Autodesk Fusion 360 part; units mm, degrees
(part 3 of 5)
  line L278 (101.5867, -7.7448) -> (99.4171, -13.4118)
  line L279 (99.4171, -13.4118) -> (84.4237, -13.4118)
  line L280 (84.4237, -13.4118) -> (91.9366, 2.5207)
  line L281 (97.7331, -10.8212) -> (98.057, -10.044)
  line L282 (98.057, -10.044) -> (90.1879, -10.044)
  line L283 (90.1879, -10.044) -> (97.5712, 5.5971)
  line L284 (97.5712, 5.5971) -> (89.864, 5.5971)
  line L285 (89.864, 5.5971) -> (89.5726, 4.8199)
  line L286 (89.5726, 4.8199) -> (96.2435, 4.8199)
  line L287 (96.2435, 4.8199) -> (88.8602, -10.8212)
  line L288 (88.8602, -10.8212) -> (97.7331, -10.8212)
extrude "Extrude1" add sketch "Sketch1" along normal blind 2 contours S0 S1 S2 L0 S3 S5 S6 L2 S7 S8 S9 S10 S11 L3 S12 S13 S14 S15 S16 S17 S18 S19 S20 S21 S22 S46 | S3 L1 S4 S5 S34 S35 S36 S37 S40 S41 S42 S43 S44 S45 S46 S47 S48 S49 S50 L5 S51 S52 S53 S54 L6 S55 S56 S57 S64 | S3 L1 S4 S5 S46 | S37 S38 S39 S40 S64 | S37 S38 S39 S40 L7 S58 S59 S60 S61 S62 S63 L8 S64 S65 S66 L9 S67 S68 S69 S70 S71 S72 S73 S74 S75 S77 S78 S79 S83 | S75 S76 S77 S83 | S75 S76 S77 S80 S81 S82 S83 S84 S85 S86 S87 S88 S89 S90 S91 S92 S93 S98 S134 S135 | S93 S94 S95 S96 S97 S98 S134 S135 | S93 S94 S95 S96 S97 S98 S106 S107 S108 S109 S110 S111 S112 S113 S114 S115 S116 S117 S118 S119 S120 S121 S122 S123 S124 S125 S126 S127 S128 S129 S130 S131 S132 S133 S134 S135 S136 S137 S138 S139 S140 S141 S142 S143 | L11 S148 S149 S150 S151 S152 L12 S153 S154 S155 S156 S157 S158 L13 S159 S160 S161 S162 S163 S164 L14 S165 S166 S167 S168 S169 S170 | S400 S401 S402 S403 S404 S405 S406 S407 S408 S409 S410 S411 S412 L177 S413 S414 S415 S416 L178 | S417 S418 L179 S419 S420 S421 L180 S422 S423 L181 S424 S425 S426 S427 S428 S429 S430 S431 S432 S433 S434 L182 S435 S436 S437 L183 S438 S439 L184 S440 | S441 S442 S443 L185 S444 S445 S446 S447 S448 S449 S450 S451 S452 S453 S454 L186 S455 S456 S457 S458 S459 L187 S460 S461 S462 S463 L188 S464 S465 S466 S467 S468 S469 S470 S471 S472 L189 | S473 S474 S475 L190 S476 S477 S478 S479 S480 S481 S482 S483 S484 S485 S486 S487 S488 S489 S490 S491 S492 S493 S494 S495 S496 S497 S498 L191 | S504 L192 S505 S506 L193 S507 S508 S509 S510 S511 S512 S513 S514 S515 S516 S517 S518 S519 S520 L194 S521 S522 S523 S524 S525 S526 S527 S528 S529 S530 S531 | S532 S533 S534 S535 S536 S537 S538 S539 L195 S540 S541 S542 S543 L196 S544 S545 S546 S547 S548 S549 S550 L197 S551 S552 S553 L198 S554 | L199 S555 S556 L200 L201 L202 S557 S558 L203 L204 | S563 S564 S565 S566 L211 L212 L213 S567 S568 S569 S570 L214 L215 L216 S571 S572 S573 S574 | L223 L224 L225 L226 L227 L228 L229 L230 L231 L232 L233 L234 | L247 L248 L249 L250 L251 L252 L253 L254 S650 L272 | L248 S614 S615 S616 S617 S618 S619 S620 S621 S622 S623 S624 S625 S626 S627 S628 S629 S630 L271 S631 S632 S633 S634 S635 S636 S637 S638 S639 S640 S641 S642 S643 S644 S645 S646 S647 S648 S649 S650 L272 | L248 S650 L272 | L266 L267 L268 | L273 L274 L275 L276 L277 L278 L279 L280 makes body 1 at (67.0712, -5.2622, 0) makes body 2 at (83.8602, -73.7685, 0) makes body 3 at (35.5259, -74.9694, 0) makes body 4 at (11.5017, -77.2089, 0) makes body 5 at (12.3957, 2.7474, 0) makes body 6 at (94.6365, -86.6871, 0) makes body 7 at (28.3473, -77.0944, 0) makes body 8 at (63.6816, -78.7236, 0) makes body 9 at (34.5713, 94.918, 0) makes body 10 at (90.4627, 77.2296, 0) makes body 11 at (98.0246, 2.0134, 0) makes body 12 at (8.1997, 1.9486, 0) makes body 13 at (62.0414, -2.1749, 0) makes body 14 at (32.4794, 0.1243, 0)
sketch "Sketch2" plane through (0, 0, 0) normal (0, 0, 1) x (1, 0, 0)
  spline S0 degree 3 poles (-205.111, 36.7973) (-205.4906, 36.9633) (-205.8582, 37.0464) (-206.214, 37.0464) knots 0 0 0 0 1 1 1 1
  spline S1 degree 3 poles (-206.214, 37.0464) (-206.5698, 37.0464) (-206.9256, 36.821) (-207.2814, 36.3703) knots 0 0 0 0 1 1 1 1
  spline S2 degree 3 poles (-207.2814, 36.3703) (-207.6372, 35.9197) (-207.8744, 35.2674) (-207.993, 34.4135) knots 0 0 0 0 1 1 1 1
  line L0 (-207.993, 34.4135) -> (-209.7719, 21.9608)
  spline S3 degree 3 poles (-209.7719, 21.9608) (-206.7833, 23.2653) (-204.8738, 24.2378) (-204.0437, 24.8783) knots 0 0 0 0 1 1 1 1
  line L1 (-204.0437, 24.8783) -> (-202.6916, 22.53)
  spline S4 degree 3 poles (-202.6916, 22.53) (-203.4032, 21.9845) (-204.2571, 21.4982) (-205.2534, 21.0713) knots 0 0 0 0 1 1 1 1
  spline S5 degree 3 poles (-205.2534, 21.0713) (-206.2496, 20.6443) (-207.2102, 20.2411) (-208.1353, 19.8616) knots 0 0 0 0 1 1 1 1
  spline S6 degree 3 poles (-208.1353, 19.8616) (-209.0603, 19.5058) (-209.7482, 19.233) (-210.1989, 19.0433) knots 0 0 0 0 1 1 1 1
  line L2 (-210.1989, 19.0433) -> (-211.373, 10.7177)
  spline S7 degree 3 poles (-211.373, 10.7177) (-211.6813, 8.4407) (-212.4997, 6.7684) (-213.8279, 5.7011) knots 0 0 0 0 1 1 1 1
  spline S8 degree 3 poles (-213.8279, 5.7011) (-215.1325, 4.6099) (-216.5794, 4.0644) (-218.1686, 4.0644) knots 0 0 0 0 1 1 1 1
  spline S9 degree 3 poles (-218.1686, 4.0644) (-219.7341, 4.0644) (-220.9794, 4.6455) (-221.9044, 5.8078) knots 0 0 0 0 1 1 1 1
  spline S10 degree 3 poles (-221.9044, 5.8078) (-222.8295, 6.9463) (-223.292, 8.2272) (-223.292, 9.6504) knots 0 0 0 0 1 1 1 1
  spline S11 degree 3 poles (-223.292, 9.6504) (-223.292, 13.3743) (-220.5643, 16.6832) (-215.1088, 19.5769) knots 0 0 0 0 1 1 1 1
  line L3 (-215.1088, 19.5769) -> (-214.753, 22.4589)
  spline S12 degree 3 poles (-214.753, 22.4589) (-214.3023, 26.5386) (-213.8398, 30.0847) (-213.3654, 33.097) knots 0 0 0 0 1 1 1 1
  spline S13 degree 3 poles (-213.3654, 33.097) (-214.7174, 32.5515) (-216.1406, 32.2787) (-217.6349, 32.2787) knots 0 0 0 0 1 1 1 1
  spline S14 degree 3 poles (-217.6349, 32.2787) (-219.1055, 32.2787) (-220.3034, 32.682) (-221.2284, 33.4884) knots 0 0 0 0 1 1 1 1
  spline S15 degree 3 poles (-221.2284, 33.4884) (-222.1298, 34.2949) (-222.5804, 35.3504) (-222.5804, 36.655) knots 0 0 0 0 1 1 1 1
  spline S16 degree 3 poles (-222.5804, 36.655) (-222.5804, 37.9596) (-222.1179, 38.9795) (-221.1928, 39.7148) knots 0 0 0 0 1 1 1 1
  spline S17 degree 3 poles (-221.1928, 39.7148) (-220.2441, 40.4738) (-219.0581, 40.8533) (-217.6349, 40.8533) knots 0 0 0 0 1 1 1 1
  spline S18 degree 3 poles (-217.6349, 40.8533) (-216.7573, 40.8533) (-215.5002, 40.5806) (-213.8635, 40.035) knots 0 0 0 0 1 1 1 1
  spline S19 degree 3 poles (-213.8635, 40.035) (-212.2031, 39.4895) (-210.9223, 39.2167) (-210.021, 39.2167) knots 0 0 0 0 1 1 1 1
  spline S20 degree 3 poles (-210.021, 39.2167) (-208.4081, 39.2167) (-207.056, 39.6318) (-205.9649, 40.462) knots 0 0 0 0 1 1 1 1
  spline S21 degree 3 poles (-205.9649, 40.462) (-205.3719, 39.6318) (-205.0755, 38.6474) (-205.0755, 37.5089) knots 0 0 0 0 1 1 1 1
  spline S22 degree 3 poles (-205.0755, 37.5089) (-205.0755, 37.2717) (-205.0873, 37.0345) (-205.111, 36.7973) knots 0 0 0 0 1 1 1 1
  spline S23 degree 3 poles (-219.0581, 35.6943) (-219.0581, 35.3385) (-218.8683, 35.0302) (-218.4888, 34.7693) knots 0 0 0 0 1 1 1 1
  spline S24 degree 3 poles (-218.4888, 34.7693) (-218.0856, 34.5084) (-217.4926, 34.3779) (-216.7099, 34.3779) knots 0 0 0 0 1 1 1 1
  spline S25 degree 3 poles (-216.7099, 34.3779) (-215.9034, 34.3779) (-214.8597, 34.7337) (-213.5789, 35.4453) knots 0 0 0 0 1 1 1 1
  spline S26 degree 3 poles (-213.5789, 35.4453) (-214.5039, 35.6588) (-215.4527, 35.896) (-216.4252, 36.1569) knots 0 0 0 0 1 1 1 1
  spline S27 degree 3 poles (-216.4252, 36.1569) (-217.3977, 36.4415) (-217.9789, 36.5838) (-218.1686, 36.5838) knots 0 0 0 0 1 1 1 1
  spline S28 degree 3 poles (-218.1686, 36.5838) (-218.7616, 36.5838) (-219.0581, 36.2873) (-219.0581, 35.6943) knots 0 0 0 0 1 1 1 1
  spline S29 degree 3 poles (-215.5002, 16.4816) (-218.892, 14.4417) (-220.588, 12.2832) (-220.588, 10.0061) knots 0 0 0 0 1 1 1 1
  spline S30 degree 3 poles (-220.588, 10.0061) (-220.588, 9.3657) (-220.422, 8.8202) (-220.0899, 8.3695) knots 0 0 0 0 1 1 1 1
  spline S31 degree 3 poles (-220.0899, 8.3695) (-219.7104, 7.8477) (-219.236, 7.5868) (-218.6667, 7.5868) knots 0 0 0 0 1 1 1 1
  spline S32 degree 3 poles (-218.6667, 7.5868) (-218.0737, 7.5868) (-217.5638, 7.7647) (-217.1368, 8.1204) knots 0 0 0 0 1 1 1 1
  spline S33 degree 3 poles (-217.1368, 8.1204) (-216.7099, 8.4762) (-216.449, 9.0455) (-216.3541, 9.8282) knots 0 0 0 0 1 1 1 1
  line L4 (-216.3541, 9.8282) -> (-215.5002, 16.4816)
  spline S34 degree 3 poles (-191.4142, 30.5709) (-192.3866, 22.8858) (-192.8729, 18.7942) (-192.8729, 18.2961) knots 0 0 0 0 1 1 1 1
  spline S35 degree 3 poles (-192.8729, 18.2961) (-192.8729, 17.3474) (-192.529, 16.8729) (-191.8411, 16.8729) knots 0 0 0 0 1 1 1 1
  spline S36 degree 3 poles (-191.8411, 16.8729) (-191.2244, 16.8729) (-190.5603, 17.288) (-189.8487, 18.1182) knots 0 0 0 0 1 1 1 1
  spline S37 degree 3 poles (-189.8487, 18.1182) (-189.1134, 18.9721) (-188.5322, 20.2411) (-188.1053, 21.9252) knots 0 0 0 0 1 1 1 1
  spline S38 degree 3 poles (-188.1053, 21.9252) (-187.3225, 21.0713) (-186.8481, 20.4071) (-186.6821, 19.9327) knots 0 0 0 0 1 1 1 1
  spline S39 degree 3 poles (-186.6821, 19.9327) (-187.2277, 17.6319) (-188.0934, 16.0072) (-189.2794, 15.0584) knots 0 0 0 0 1 1 1 1
  spline S40 degree 3 poles (-189.2794, 15.0584) (-190.4654, 14.1096) (-191.6869, 13.6352) (-192.9441, 13.6352) knots 0 0 0 0 1 1 1 1
  spline S41 degree 3 poles (-192.9441, 13.6352) (-195.0077, 13.6352) (-196.3952, 14.4298) (-197.1068, 16.019) knots 0 0 0 0 1 1 1 1
  spline S42 degree 3 poles (-197.1068, 16.019) (-198.3402, 14.4298) (-199.9887, 13.6352) (-202.0523, 13.6352) knots 0 0 0 0 1 1 1 1
  spline S43 degree 3 poles (-202.0523, 13.6352) (-203.7601, 13.6352) (-205.0766, 14.0622) (-206.0016, 14.9161) knots 0 0 0 0 1 1 1 1
  spline S44 degree 3 poles (-206.0016, 14.9161) (-206.9267, 15.77) (-207.3892, 16.8848) (-207.3892, 18.2605) knots 0 0 0 0 1 1 1 1
  spline S45 degree 3 poles (-207.3892, 18.2605) (-207.3892, 18.5926) (-207.3299, 19.1737) (-207.2113, 20.0039) knots 0 0 0 0 1 1 1 1
  spline S46 degree 3 poles (-207.2113, 20.0039) (-206.6657, 24.4157) (-206.2507, 27.9262) (-205.9661, 30.5353) knots 0 0 0 0 1 1 1 1
  spline S47 degree 3 poles (-205.9661, 30.5353) (-205.2307, 30.7963) (-204.5547, 30.9267) (-203.938, 30.9267) knots 0 0 0 0 1 1 1 1
  spline S48 degree 3 poles (-203.938, 30.9267) (-203.3213, 30.9267) (-202.8588, 30.903) (-202.5504, 30.8556) knots 0 0 0 0 1 1 1 1
  spline S49 degree 3 poles (-202.5504, 30.8556) (-202.2421, 30.8081) (-201.9456, 30.6302) (-201.661, 30.3219) knots 0 0 0 0 1 1 1 1
  spline S50 degree 3 poles (-201.661, 30.3219) (-201.3763, 30.0136) (-201.234, 29.5747) (-201.234, 29.0054) knots 0 0 0 0 1 1 1 1
  line L5 (-201.234, 29.0054) -> (-202.4081, 19.9327)
  spline S51 degree 3 poles (-202.4081, 19.9327) (-202.4556, 19.6481) (-202.4793, 19.3872) (-202.4793, 19.15) knots 0 0 0 0 1 1 1 1
  spline S52 degree 3 poles (-202.4793, 19.15) (-202.4793, 17.7506) (-201.8389, 17.0508) (-200.558, 17.0508) knots 0 0 0 0 1 1 1 1
  spline S53 degree 3 poles (-200.558, 17.0508) (-199.372, 17.0508) (-198.3877, 17.632) (-197.6049, 18.7942) knots 0 0 0 0 1 1 1 1
  spline S54 degree 3 poles (-197.6049, 18.7942) (-197.6049, 19.0552) (-197.5812, 19.4702) (-197.5338, 20.0395) knots 0 0 0 0 1 1 1 1
  line L6 (-197.5338, 20.0395) -> (-196.3597, 29.5035)
  spline S55 degree 3 poles (-196.3597, 29.5035) (-196.1936, 29.9068) (-195.8378, 30.2389) (-195.2923, 30.4998) knots 0 0 0 0 1 1 1 1
  spline S56 degree 3 poles (-195.2923, 30.4998) (-194.7467, 30.7844) (-194.0707, 30.9267) (-193.2643, 30.9267) knots 0 0 0 0 1 1 1 1
  spline S57 degree 3 poles (-193.2643, 30.9267) (-192.4341, 30.9267) (-191.8174, 30.8081) (-191.4142, 30.5709) knots 0 0 0 0 1 1 1 1
  line L7 (-179.5365, 17.8691) -> (-178.6826, 25.7322)
  spline S58 degree 3 poles (-178.6826, 25.7322) (-178.6826, 26.3726) (-178.8487, 26.9063) (-179.1808, 27.3332) knots 0 0 0 0 1 1 1 1
  spline S59 degree 3 poles (-179.1808, 27.3332) (-179.5128, 27.7602) (-180.0465, 27.9736) (-180.7818, 27.9736) knots 0 0 0 0 1 1 1 1
  spline S60 degree 3 poles (-180.7818, 27.9736) (-181.5171, 27.9736) (-182.1457, 27.6772) (-182.6675, 27.0842) knots 0 0 0 0 1 1 1 1
  spline S61 degree 3 poles (-182.6675, 27.0842) (-183.1656, 26.5149) (-183.5333, 25.7559) (-183.7705, 24.8071) knots 0 0 0 0 1 1 1 1
  spline S62 degree 3 poles (-183.7705, 24.8071) (-183.9365, 23.4551) (-184.1855, 21.4745) (-184.5176, 18.8654) knots 0 0 0 0 1 1 1 1
  spline S63 degree 3 poles (-184.5176, 18.8654) (-184.8497, 16.28) (-185.0632, 14.5959) (-185.1581, 13.8131) knots 0 0 0 0 1 1 1 1
  line L8 (-185.1581, 13.8131) -> (-189.8901, 13.8131)
  spline S64 degree 3 poles (-189.8901, 13.8131) (-188.1823, 28.3532) (-187.1505, 37.2835) (-186.7947, 40.6043) knots 0 0 0 0 1 1 1 1
  spline S65 degree 3 poles (-186.7947, 40.6043) (-186.2966, 40.794) (-185.6206, 40.8889) (-184.7667, 40.8889) knots 0 0 0 0 1 1 1 1
  spline S66 degree 3 poles (-184.7667, 40.8889) (-182.9166, 40.8889) (-181.9915, 40.3434) (-181.9915, 39.2523) knots 0 0 0 0 1 1 1 1
  line L9 (-181.9915, 39.2523) -> (-181.9915, 39.0388)
  spline S67 degree 3 poles (-181.9915, 39.0388) (-182.3947, 35.3149) (-182.8217, 32.0416) (-183.2724, 29.2189) knots 0 0 0 0 1 1 1 1
  spline S68 degree 3 poles (-183.2724, 29.2189) (-182.0152, 30.3574) (-180.592, 30.9267) (-179.0029, 30.9267) knots 0 0 0 0 1 1 1 1
  spline S69 degree 3 poles (-179.0029, 30.9267) (-177.4136, 30.9267) (-176.1565, 30.5235) (-175.2315, 29.717) knots 0 0 0 0 1 1 1 1
  spline S70 degree 3 poles (-175.2315, 29.717) (-174.3064, 28.9106) (-173.8439, 27.8906) (-173.8439, 26.6572) knots 0 0 0 0 1 1 1 1
  spline S71 degree 3 poles (-173.8439, 26.6572) (-173.8439, 26.3252) (-173.915, 25.7085) (-174.0573, 24.8071) knots 0 0 0 0 1 1 1 1
  spline S72 degree 3 poles (-174.0573, 24.8071) (-174.6029, 21.2492) (-174.8757, 19.1619) (-174.8757, 18.5452) knots 0 0 0 0 1 1 1 1
  spline S73 degree 3 poles (-174.8757, 18.5452) (-174.8757, 17.4304) (-174.508, 16.8729) (-173.7727, 16.8729) knots 0 0 0 0 1 1 1 1
  spline S74 degree 3 poles (-173.7727, 16.8729) (-173.156, 16.8729) (-172.5037, 17.2762) (-171.816, 18.0826) knots 0 0 0 0 1 1 1 1
  spline S75 degree 3 poles (-171.816, 18.0826) (-171.1044, 18.9128) (-170.5352, 20.1818) (-170.1082, 21.8896) knots 0 0 0 0 1 1 1 1
  spline S76 degree 3 poles (-170.1082, 21.8896) (-169.3016, 21.0357) (-168.8152, 20.3597) (-168.6495, 19.8616) knots 0 0 0 0 1 1 1 1
  spline S77 degree 3 poles (-168.6495, 19.8616) (-169.8825, 15.7344) (-172.0651, 13.6708) (-175.1959, 13.6708) knots 0 0 0 0 1 1 1 1
  spline S78 degree 3 poles (-175.1959, 13.6708) (-176.6665, 13.6708) (-177.7576, 14.1215) (-178.4692, 15.0228) knots 0 0 0 0 1 1 1 1
  spline S79 degree 3 poles (-178.4692, 15.0228) (-179.1808, 15.9241) (-179.5365, 16.8729) (-179.5365, 17.8691) knots 0 0 0 0 1 1 1 1
  spline S80 degree 3 poles (-155.7317, 13.6352) (-157.9137, 13.6352) (-159.3607, 14.3942) (-160.0723, 15.9123) knots 0 0 0 0 1 1 1 1
  spline S81 degree 3 poles (-160.0723, 15.9123) (-161.3054, 14.3705) (-162.8948, 13.5996) (-164.8399, 13.5996) knots 0 0 0 0 1 1 1 1
  spline S82 degree 3 poles (-164.8399, 13.5996) (-166.7612, 13.5996) (-168.3857, 14.2519) (-169.7143, 15.5565) knots 0 0 0 0 1 1 1 1
  spline S83 degree 3 poles (-169.7143, 15.5565) (-171.0185, 16.8611) (-171.6712, 18.5807) (-171.6712, 20.7155) knots 0 0 0 0 1 1 1 1
  spline S84 degree 3 poles (-171.6712, 20.7155) (-171.6712, 23.8228) (-170.7578, 26.3014) (-168.9316, 28.1515) knots 0 0 0 0 1 1 1 1
  spline S85 degree 3 poles (-168.9316, 28.1515) (-167.1048, 30.0017) (-164.7922, 30.9267) (-161.9936, 30.9267) knots 0 0 0 0 1 1 1 1
  spline S86 degree 3 poles (-161.9936, 30.9267) (-161.9225, 30.9267) (-161.8513, 30.9267) (-161.7801, 30.9267) knots 0 0 0 0 1 1 1 1
  spline S87 degree 3 poles (-161.7801, 30.9267) (-160.5938, 30.9267) (-159.5031, 30.7251) (-158.5068, 30.3219) knots 0 0 0 0 1 1 1 1
  spline S88 degree 3 poles (-158.5068, 30.3219) (-157.8664, 30.7251) (-157.0954, 30.9267) (-156.1942, 30.9267) knots 0 0 0 0 1 1 1 1
  spline S89 degree 3 poles (-156.1942, 30.9267) (-155.2691, 30.9267) (-154.6048, 30.8081) (-154.2018, 30.5709) knots 0 0 0 0 1 1 1 1
  spline S90 degree 3 poles (-154.2018, 30.5709) (-154.4152, 28.8157) (-154.6404, 27.0842) (-154.8778, 25.3764) knots 0 0 0 0 1 1 1 1
  spline S91 degree 3 poles (-154.8778, 25.3764) (-155.1146, 23.6923) (-155.2808, 22.4944) (-155.3759, 21.7829) knots 0 0 0 0 1 1 1 1
  spline S92 degree 3 poles (-155.3759, 21.7829) (-155.5894, 20.17) (-155.6961, 19.0077) (-155.6961, 18.2961) knots 0 0 0 0 1 1 1 1
  spline S93 degree 3 poles (-155.6961, 18.2961) (-155.6961, 17.3474) (-155.3164, 16.8729) (-154.5576, 16.8729) knots 0 0 0 0 1 1 1 1
  spline S94 degree 3 poles (-154.5576, 16.8729) (-153.9644, 16.8729) (-153.3357, 17.2643) (-152.6719, 18.047) knots 0 0 0 0 1 1 1 1
  spline S95 degree 3 poles (-152.6719, 18.047) (-152.0075, 18.8535) (-151.4266, 20.1106) (-150.9285, 21.8184) knots 0 0 0 0 1 1 1 1
  spline S96 degree 3 poles (-150.9285, 21.8184) (-150.2403, 21.2018) (-149.7661, 20.5139) (-149.5053, 19.7548) knots 0 0 0 0 1 1 1 1
  spline S97 degree 3 poles (-149.5053, 19.7548) (-150.193, 17.5015) (-151.1181, 15.9123) (-152.2805, 14.9872) knots 0 0 0 0 1 1 1 1
  spline S98 degree 3 poles (-152.2805, 14.9872) (-153.4424, 14.0859) (-154.5931, 13.6352) (-155.7317, 13.6352) knots 0 0 0 0 1 1 1 1
  spline S99 degree 3 poles (-161.4599, 28.1515) (-162.9776, 28.1515) (-164.1873, 27.5704) (-165.089, 26.4082) knots 0 0 0 0 1 1 1 1
  spline S100 degree 3 poles (-165.089, 26.4082) (-165.9663, 25.2696) (-166.4883, 23.5618) (-166.6545, 21.2848) knots 0 0 0 0 1 1 1 1
  spline S101 degree 3 poles (-166.6545, 21.2848) (-166.6779, 21.0713) (-166.6901, 20.8697) (-166.6901, 20.6799) knots 0 0 0 0 1 1 1 1
  spline S102 degree 3 poles (-166.6901, 20.6799) (-166.6901, 19.5177) (-166.4171, 18.5926) (-165.8717, 17.9047) knots 0 0 0 0 1 1 1 1
  spline S103 degree 3 poles (-165.8717, 17.9047) (-165.3025, 17.2169) (-164.5787, 16.8729) (-163.7014, 16.8729) knots 0 0 0 0 1 1 1 1
  spline S104 degree 3 poles (-163.7014, 16.8729) (-162.2071, 16.8729) (-161.0802, 17.9285) (-160.3214, 20.0395) knots 0 0 0 0 1 1 1 1
  line L10 (-160.3214, 20.0395) -> (-159.4675, 27.7246)
  spline S105 degree 3 poles (-159.4675, 27.7246) (-160.1552, 28.0092) (-160.8195, 28.1515) (-161.4599, 28.1515) knots 0 0 0 0 1 1 1 1
  spline S106 degree 3 poles (-137.2, 24.7004) (-135.326, 23.3247) (-134.3892, 21.6999) (-134.3892, 19.826) knots 0 0 0 0 1 1 1 1
  spline S107 degree 3 poles (-134.3892, 19.826) (-134.3892, 17.9521) (-135.1247, 16.446) (-136.5951, 15.3074) knots 0 0 0 0 1 1 1 1
  spline S108 degree 3 poles (-136.5951, 15.3074) (-138.0656, 14.1689) (-139.9157, 13.5996) (-142.1455, 13.5996) knots 0 0 0 0 1 1 1 1
  spline S109 degree 3 poles (-142.1455, 13.5996) (-143.5926, 13.5996) (-144.8022, 13.9554) (-145.7746, 14.667) knots 0 0 0 0 1 1 1 1
  spline S110 degree 3 poles (-145.7746, 14.667) (-146.7235, 15.4023) (-147.1977, 16.3037) (-147.1977, 17.371) knots 0 0 0 0 1 1 1 1
  spline S111 degree 3 poles (-147.1977, 17.371) (-147.1977, 18.4384) (-146.8419, 19.2805) (-146.1304, 19.8972) knots 0 0 0 0 1 1 1 1
  spline S112 degree 3 poles (-146.1304, 19.8972) (-145.4188, 20.5376) (-144.5293, 20.929) (-143.4619, 21.0713) knots 0 0 0 0 1 1 1 1
  spline S113 degree 3 poles (-143.4619, 21.0713) (-143.96, 20.3597) (-144.2091, 19.6718) (-144.2091, 19.0077) knots 0 0 0 0 1 1 1 1
  spline S114 degree 3 poles (-144.2091, 19.0077) (-144.2091, 18.3673) (-143.9839, 17.8455) (-143.5331, 17.4422) knots 0 0 0 0 1 1 1 1
  spline S115 degree 3 poles (-143.5331, 17.4422) (-143.0822, 17.039) (-142.513, 16.8374) (-141.8253, 16.8374) knots 0 0 0 0 1 1 1 1
  spline S116 degree 3 poles (-141.8253, 16.8374) (-141.1376, 16.8374) (-140.5683, 17.0864) (-140.1175, 17.5845) knots 0 0 0 0 1 1 1 1
  spline S117 degree 3 poles (-140.1175, 17.5845) (-139.6666, 18.1064) (-139.4415, 18.6994) (-139.4415, 19.3635) knots 0 0 0 0 1 1 1 1
  spline S118 degree 3 poles (-139.4415, 19.3635) (-139.4415, 20.4546) (-139.9513, 21.4271) (-140.9714, 22.281) knots 0 0 0 0 1 1 1 1
  spline S119 degree 3 poles (-140.9714, 22.281) (-141.5879, 22.7791) (-142.2522, 23.2416) (-142.9638, 23.6686) knots 0 0 0 0 1 1 1 1
  spline S120 degree 3 poles (-142.9638, 23.6686) (-143.6754, 24.1192) (-144.0551, 24.3565) (-144.1023, 24.3801) knots 0 0 0 0 1 1 1 1
  spline S121 degree 3 poles (-144.1023, 24.3801) (-144.1974, 24.4513) (-144.2919, 24.5106) (-144.387, 24.558) knots 0 0 0 0 1 1 1 1
  spline S122 degree 3 poles (-144.387, 24.558) (-144.8139, 24.0599) (-145.4305, 23.3721) (-146.2371, 22.4944) knots 0 0 0 0 1 1 1 1
  spline S123 degree 3 poles (-146.2371, 22.4944) (-147.0437, 21.6405) (-147.6842, 20.9527) (-148.1584, 20.4309) knots 0 0 0 0 1 1 1 1
  spline S124 degree 3 poles (-148.1584, 20.4309) (-149.4865, 18.9839) (-150.2337, 17.7743) (-150.3999, 16.8018) knots 0 0 0 0 1 1 1 1
  spline S125 degree 3 poles (-150.3999, 16.8018) (-150.4471, 16.612) (-150.471, 16.2444) (-150.471, 15.6988) knots 0 0 0 0 1 1 1 1
  spline S126 degree 3 poles (-150.471, 15.6988) (-150.471, 15.177) (-150.317, 14.6314) (-150.0085, 14.0622) knots 0 0 0 0 1 1 1 1
  spline S127 degree 3 poles (-150.0085, 14.0622) (-149.6766, 13.4929) (-149.2852, 13.066) (-148.8344, 12.7813) knots 0 0 0 0 1 1 1 1
  spline S128 degree 3 poles (-148.8344, 12.7813) (-148.3835, 12.4967) (-147.9449, 12.2714) (-147.518, 12.1053) knots 0 0 0 0 1 1 1 1
  spline S129 degree 3 poles (-147.518, 12.1053) (-147.0671, 11.9156) (-146.6879, 11.7851) (-146.3794, 11.7139) knots 0 0 0 0 1 1 1 1
  spline S130 degree 3 poles (-146.3794, 11.7139) (-146.0475, 11.6428) (-145.8813, 11.5954) (-145.8813, 11.5716) knots 0 0 0 0 1 1 1 1
  spline S131 degree 3 poles (-145.8813, 11.5716) (-145.8813, 11.4056) (-146.1421, 11.2158) (-146.6641, 11.0024) knots 0 0 0 0 1 1 1 1
  spline S132 degree 3 poles (-146.6641, 11.0024) (-147.6364, 10.6466) (-148.6565, 10.4687) (-149.7239, 10.4687) knots 0 0 0 0 1 1 1 1
  spline S133 degree 3 poles (-149.7239, 10.4687) (-150.7674, 10.4687) (-151.7875, 10.8482) (-152.7837, 11.6072) knots 0 0 0 0 1 1 1 1
  spline S134 degree 3 poles (-152.7837, 11.6072) (-154.1357, 12.6508) (-154.8117, 14.0385) (-154.8117, 15.77) knots 0 0 0 0 1 1 1 1
  spline S135 degree 3 poles (-154.8117, 15.77) (-154.8117, 16.8374) (-154.5387, 17.8929) (-153.9934, 18.9365) knots 0 0 0 0 1 1 1 1
  spline S136 degree 3 poles (-153.9934, 18.9365) (-153.021, 20.7866) (-150.744, 23.3247) (-147.1622, 26.5505) knots 0 0 0 0 1 1 1 1
  spline S137 degree 3 poles (-147.1622, 26.5505) (-148.04, 27.4281) (-148.4786, 28.365) (-148.4786, 29.3612) knots 0 0 0 0 1 1 1 1
  spline S138 degree 3 poles (-148.4786, 29.3612) (-148.4786, 30.3574) (-148.1111, 31.1995) (-147.3756, 31.8874) knots 0 0 0 0 1 1 1 1
  spline S139 degree 3 poles (-147.3756, 31.8874) (-146.6168, 32.5753) (-145.7273, 32.9192) (-144.7072, 32.9192) knots 0 0 0 0 1 1 1 1
  spline S140 degree 3 poles (-144.7072, 32.9192) (-143.7821, 32.9192) (-142.9755, 32.5515) (-142.2878, 31.8162) knots 0 0 0 0 1 1 1 1
  spline S141 degree 3 poles (-142.2878, 31.8162) (-141.837, 31.3181) (-141.6118, 30.6896) (-141.6118, 29.9305) knots 0 0 0 0 1 1 1 1
  spline S142 degree 3 poles (-141.6118, 29.9305) (-141.6118, 29.1715) (-141.8609, 28.3176) (-142.359, 27.3688) knots 0 0 0 0 1 1 1 1
  spline S143 degree 3 poles (-142.359, 27.3688) (-139.8212, 26.2303) (-138.1012, 25.3408) (-137.2, 24.7004) knots 0 0 0 0 1 1 1 1
  spline S144 degree 3 poles (-144.9207, 28.7208) (-144.3514, 29.3138) (-144.0668, 29.7408) (-144.0668, 30.0017) knots 0 0 0 0 1 1 1 1
  spline S145 degree 3 poles (-144.0668, 30.0017) (-144.0668, 30.5947) (-144.3275, 30.9149) (-144.8495, 30.9623) knots 0 0 0 0 1 1 1 1
  spline S146 degree 3 poles (-144.8495, 30.9623) (-145.4427, 30.9623) (-145.739, 30.6302) (-145.739, 29.9661) knots 0 0 0 0 1 1 1 1
  spline S147 degree 3 poles (-145.739, 29.9661) (-145.739, 29.5629) (-145.466, 29.1478) (-144.9207, 28.7208) knots 0 0 0 0 1 1 1 1
  line L11 (-124.331, 13.4928) -> (-134.222, 13.7063)
  spline S148 degree 3 poles (-134.222, 13.7063) (-134.5305, 13.7063) (-134.6845, 14.1214) (-134.6845, 14.9516) knots 0 0 0 0 1 1 1 1
  spline S149 degree 3 poles (-134.6845, 14.9516) (-134.6845, 15.8055) (-134.5066, 16.4696) (-134.1508, 16.944) knots 0 0 0 0 1 1 1 1
  spline S150 degree 3 poles (-134.1508, 16.944) (-133.7951, 17.8928) (-132.8105, 19.2804) (-131.1978, 21.1068) knots 0 0 0 0 1 1 1 1
  spline S151 degree 3 poles (-131.1978, 21.1068) (-130.6758, 21.6998) (-129.7034, 22.7671) (-128.2803, 24.3089) knots 0 0 0 0 1 1 1 1
  spline S152 degree 3 poles (-128.2803, 24.3089) (-126.8571, 25.8507) (-125.9204, 26.9062) (-125.4695, 27.4754) knots 0 0 0 0 1 1 1 1
  line L12 (-125.4695, 27.4754) -> (-127.3552, 27.5822)
  spline S153 degree 3 poles (-127.3552, 27.5822) (-127.711, 26.7283) (-128.233, 26.0286) (-128.9207, 25.483) knots 0 0 0 0 1 1 1 1
  spline S154 degree 3 poles (-128.9207, 25.483) (-129.585, 24.9612) (-130.3322, 24.7003) (-131.1622, 24.7003) knots 0 0 0 0 1 1 1 1
  spline S155 degree 3 poles (-131.1622, 24.7003) (-132.1111, 24.7003) (-132.8817, 24.973) (-133.4748, 25.5186) knots 0 0 0 0 1 1 1 1
  spline S156 degree 3 poles (-133.4748, 25.5186) (-134.068, 26.0878) (-134.3643, 26.8706) (-134.3643, 27.8668) knots 0 0 0 0 1 1 1 1
  spline S157 degree 3 poles (-134.3643, 27.8668) (-134.3643, 28.863) (-134.0202, 29.6577) (-133.3325, 30.2506) knots 0 0 0 0 1 1 1 1
  spline S158 degree 3 poles (-133.3325, 30.2506) (-132.6448, 30.8436) (-131.6959, 31.1401) (-130.4862, 31.1401) knots 0 0 0 0 1 1 1 1
  line L13 (-130.4862, 31.1401) -> (-120.5952, 30.9266)
  spline S159 degree 3 poles (-120.5952, 30.9266) (-120.2866, 30.9266) (-120.1326, 30.5234) (-120.1326, 29.7169) knots 0 0 0 0 1 1 1 1
  spline S160 degree 3 poles (-120.1326, 29.7169) (-120.1326, 28.8868) (-120.2866, 28.2463) (-120.5952, 27.7956) knots 0 0 0 0 1 1 1 1
  spline S161 degree 3 poles (-120.5952, 27.7956) (-120.8798, 27.2739) (-121.2951, 26.7164) (-121.8404, 26.1234) knots 0 0 0 0 1 1 1 1
  spline S162 degree 3 poles (-121.8404, 26.1234) (-122.3624, 25.5542) (-123.133, 24.7833) (-124.1531, 23.8108) knots 0 0 0 0 1 1 1 1
  spline S163 degree 3 poles (-124.1531, 23.8108) (-125.1732, 22.862) (-125.8848, 22.186) (-126.2878, 21.7828) knots 0 0 0 0 1 1 1 1
  spline S164 degree 3 poles (-126.2878, 21.7828) (-127.8772, 20.1936) (-129.063, 18.6637) (-129.8458, 17.193) knots 0 0 0 0 1 1 1 1
  line L14 (-129.8458, 17.193) -> (-127.462, 17.0507)
  spline S165 degree 3 poles (-127.462, 17.0507) (-127.1062, 17.9046) (-126.5964, 18.5925) (-125.9321, 19.1143) knots 0 0 0 0 1 1 1 1
  spline S166 degree 3 poles (-125.9321, 19.1143) (-125.2443, 19.6599) (-124.485, 19.9326) (-123.655, 19.9326) knots 0 0 0 0 1 1 1 1
  spline S167 degree 3 poles (-123.655, 19.9326) (-122.706, 19.9326) (-121.9355, 19.648) (-121.3423, 19.0787) knots 0 0 0 0 1 1 1 1
  spline S168 degree 3 poles (-121.3423, 19.0787) (-120.7492, 18.5332) (-120.4529, 17.7623) (-120.4529, 16.7661) knots 0 0 0 0 1 1 1 1
  spline S169 degree 3 poles (-120.4529, 16.7661) (-120.4529, 15.7699) (-120.7969, 14.9753) (-121.4846, 14.3823) knots 0 0 0 0 1 1 1 1
  spline S170 degree 3 poles (-121.4846, 14.3823) (-122.1723, 13.7893) (-123.1213, 13.4928) (-124.331, 13.4928) knots 0 0 0 0 1 1 1 1
  spline S171 degree 3 poles (-130.7708, 27.8312) (-131.6008, 27.8312) (-132.0161, 27.5585) (-132.0161, 27.0129) knots 0 0 0 0 1 1 1 1
  spline S172 degree 3 poles (-132.0161, 27.0129) (-132.0161, 26.4674) (-131.7076, 26.1946) (-131.091, 26.1946) knots 0 0 0 0 1 1 1 1
  spline S173 degree 3 poles (-131.091, 26.1946) (-130.166, 26.1946) (-129.4305, 26.6927) (-128.8851, 27.6889) knots 0 0 0 0 1 1 1 1
  line L15 (-128.8851, 27.6889) -> (-130.3439, 27.7956)
  spline S174 degree 3 poles (-130.3439, 27.7956) (-130.4862, 27.8194) (-130.6285, 27.8312) (-130.7708, 27.8312) knots 0 0 0 0 1 1 1 1
  spline S175 degree 3 poles (-124.0463, 16.8017) (-123.2163, 16.8017) (-122.8011, 17.0745) (-122.8011, 17.62) knots 0 0 0 0 1 1 1 1
  spline S176 degree 3 poles (-122.8011, 17.62) (-122.8011, 18.1656) (-123.1096, 18.4383) (-123.7261, 18.4383) knots 0 0 0 0 1 1 1 1
  spline S177 degree 3 poles (-123.7261, 18.4383) (-124.6512, 18.4383) (-125.3867, 17.9402) (-125.9321, 16.944) knots 0 0 0 0 1 1 1 1
  line L16 (-125.9321, 16.944) -> (-124.4733, 16.8372)
  spline S178 degree 3 poles (-124.4733, 16.8372) (-124.331, 16.8136) (-124.1887, 16.8017) (-124.0463, 16.8017) knots 0 0 0 0 1 1 1 1
  spline S179 degree 3 poles (-131.3299, 16.1004) (-133.9729, 15.897) (-135.3961, 18.8111) (-135.6503, 19.9124) knots 0 0 0 0 1 1 1 1
  spline S180 degree 3 poles (-135.6503, 19.9124) (-137.4292, 18.8959) (-140.3081, 13.272) (-138.4458, 14.5755) knots 0 0 0 0 1 1 1 1
  spline S181 degree 3 poles (-138.4458, 14.5755) (-135.9044, 16.3545) (-133.702, 14.8297) (-133.1089, 14.0673) knots 0 0 0 0 1 1 1 1
  line L17 (-133.1089, 14.0673) -> (-131.8382, 14.5755)
  spline S182 degree 3 poles (-131.8382, 14.5755) (-130.7368, 15.0838) (-128.6869, 16.3037) (-131.3299, 16.1004) knots 0 0 0 0 1 1 1 1
extrude "Extrude2" add sketch "Sketch2" along normal blind 3 separate body makes body 15
sketch "Sketch3" plane through (0, 0, 0) normal (0, 0, 1) x (1, 0, 0)
  spline S0 degree 3 poles (220.0582, 22.2708) (220.0582, 23.1141) (220.431, 23.8109) (221.1767, 24.3613) knots 0 0 0 0 1 1 1 1
  spline S1 degree 3 poles (221.1767, 24.3613) (221.9223, 24.9205) (222.9076, 25.2001) (224.1325, 25.2001) knots 0 0 0 0 1 1 1 1
  spline S2 degree 3 poles (224.1325, 25.2001) (224.7805, 25.2001) (225.3619, 25.1335) (225.8768, 25.0004) knots 0 0 0 0 1 1 1 1
  spline S3 degree 3 poles (225.8768, 25.0004) (226.3916, 24.8761) (226.7999, 24.7163) (227.1017, 24.521) knots 0 0 0 0 1 1 1 1
  spline S4 degree 3 poles (227.1017, 24.521) (227.4035, 24.3257) (227.6565, 24.0994) (227.8607, 23.842) knots 0 0 0 0 1 1 1 1
  spline S5 degree 3 poles (227.8607, 23.842) (228.198, 23.3982) (228.3622, 22.9011) (228.3533, 22.3507) knots 0 0 0 0 1 1 1 1
  spline S6 degree 3 poles (228.3533, 22.3507) (228.3533, 21.8093) (228.1403, 21.3255) (227.7142, 20.8994) knots 0 0 0 0 1 1 1 1
  spline S7 degree 3 poles (227.7142, 20.8994) (227.2881, 20.4733) (226.7733, 20.2514) (226.1697, 20.2337) knots 0 0 0 0 1 1 1 1
  spline S8 degree 3 poles (226.1697, 20.2337) (226.9242, 20.1804) (227.5766, 19.9319) (228.127, 19.4881) knots 0 0 0 0 1 1 1 1
  spline S9 degree 3 poles (228.127, 19.4881) (228.6862, 19.0442) (228.9658, 18.485) (228.9658, 17.8104) knots 0 0 0 0 1 1 1 1
  spline S10 degree 3 poles (228.9658, 17.8104) (228.9658, 16.9228) (228.624, 16.2304) (227.9405, 15.7333) knots 0 0 0 0 1 1 1 1
  spline S11 degree 3 poles (227.9405, 15.7333) (227.257, 15.2362) (226.4227, 14.9877) (225.4374, 14.9877) knots 0 0 0 0 1 1 1 1
  spline S12 degree 3 poles (225.4374, 14.9877) (224.4609, 14.9877) (223.7952, 15.1164) (223.4402, 15.3738) knots 0 0 0 0 1 1 1 1
  line L0 (223.4402, 15.3738) -> (223.8529, 16.4922)
  spline S13 degree 3 poles (223.8529, 16.4922) (224.2435, 16.2881) (224.6962, 16.186) (225.211, 16.186) knots 0 0 0 0 1 1 1 1
  spline S14 degree 3 poles (225.211, 16.186) (225.7347, 16.186) (226.1608, 16.3369) (226.4892, 16.6387) knots 0 0 0 0 1 1 1 1
  spline S15 degree 3 poles (226.4892, 16.6387) (226.8177, 16.9494) (226.9819, 17.3577) (226.9819, 17.8637) knots 0 0 0 0 1 1 1 1
  spline S16 degree 3 poles (226.9819, 17.8637) (226.9819, 18.3696) (226.7555, 18.7957) (226.3028, 19.1419) knots 0 0 0 0 1 1 1 1
  spline S17 degree 3 poles (226.3028, 19.1419) (225.859, 19.4881) (225.251, 19.6611) (224.4787, 19.6611) knots 0 0 0 0 1 1 1 1
  line L1 (224.4787, 19.6611) -> (224.5985, 20.6464)
  spline S18 degree 3 poles (224.5985, 20.6464) (225.1311, 20.6464) (225.5794, 20.7707) (225.9433, 21.0193) knots 0 0 0 0 1 1 1 1
  spline S19 degree 3 poles (225.9433, 21.0193) (226.3161, 21.2767) (226.507, 21.6584) (226.5159, 22.1643) knots 0 0 0 0 1 1 1 1
  spline S20 degree 3 poles (226.5159, 22.1643) (226.5336, 22.6703) (226.3073, 23.0964) (225.8368, 23.4425) knots 0 0 0 0 1 1 1 1
  spline S21 degree 3 poles (225.8368, 23.4425) (225.3309, 23.8065) (224.6385, 23.9884) (223.7597, 23.9884) knots 0 0 0 0 1 1 1 1
  spline S22 degree 3 poles (223.7597, 23.9884) (223.1827, 23.9884) (222.6191, 23.8375) (222.0687, 23.5357) knots 0 0 0 0 1 1 1 1
  spline S23 degree 3 poles (222.0687, 23.5357) (221.5184, 23.2428) (221.2432, 22.8478) (221.2432, 22.3507) knots 0 0 0 0 1 1 1 1
  spline S24 degree 3 poles (221.2432, 22.3507) (221.2432, 22.1111) (221.3409, 21.9069) (221.5362, 21.7382) knots 0 0 0 0 1 1 1 1
  spline S25 degree 3 poles (221.5362, 21.7382) (221.7314, 21.5785) (222.375, 21.4942) (222.6945, 21.4586) knots 0 0 0 0 1 1 1 1
  line L2 (222.6945, 21.4586) -> (222.6945, 20.4467)
  spline S26 degree 3 poles (222.6945, 20.4467) (222.0199, 20.4733) (220.9681, 20.6775) (220.6041, 21.0326) knots 0 0 0 0 1 1 1 1
  spline S27 degree 3 poles (220.6041, 21.0326) (220.2402, 21.3876) (220.0582, 21.8004) (220.0582, 22.2708) knots 0 0 0 0 1 1 1 1
  spline S28 degree 3 poles (223.8662, 17.624) (223.7242, 16.6742) (223.449, 15.9996) (223.0407, 15.6002) knots 0 0 0 0 1 1 1 1
  spline S29 degree 3 poles (223.0407, 15.6002) (222.6324, 15.2096) (222.1531, 15.0143) (221.6027, 15.0143) knots 0 0 0 0 1 1 1 1
  spline S30 degree 3 poles (221.6027, 15.0143) (221.0524, 15.0143) (220.6352, 15.1563) (220.3511, 15.4404) knots 0 0 0 0 1 1 1 1
  spline S31 degree 3 poles (220.3511, 15.4404) (220.0671, 15.7244) (219.9251, 16.0884) (219.9251, 16.5322) knots 0 0 0 0 1 1 1 1
  spline S32 degree 3 poles (219.9251, 16.5322) (219.9251, 17.5796) (220.7195, 18.4717) (222.3084, 19.2084) knots 0 0 0 0 1 1 1 1
  spline S33 degree 3 poles (222.3084, 19.2084) (222.3528, 19.5813) (222.4149, 20.0828) (222.4948, 20.713) knots 0 0 0 0 1 1 1 1
  spline S34 degree 3 poles (222.4948, 20.713) (222.5836, 21.3521) (222.6501, 21.867) (222.6945, 22.2575) knots 0 0 0 0 1 1 1 1
  spline S35 degree 3 poles (222.6945, 22.2575) (222.7478, 22.6481) (222.7833, 22.9055) (222.8011, 23.0298) knots 0 0 0 0 1 1 1 1
  spline S36 degree 3 poles (222.8011, 23.0298) (223.165, 23.2606) (223.5866, 23.376) (224.066, 23.376) knots 0 0 0 0 1 1 1 1
  spline S37 degree 3 poles (224.066, 23.376) (224.2879, 23.376) (224.5009, 23.3538) (224.7051, 23.3094) knots 0 0 0 0 1 1 1 1
  line L3 (224.7051, 23.3094) -> (223.8662, 17.624)
  spline S38 degree 3 poles (220.9104, 16.7053) (220.9104, 16.3857) (221.0613, 16.2259) (221.3631, 16.2259) knots 0 0 0 0 1 1 1 1
  spline S39 degree 3 poles (221.3631, 16.2259) (221.4873, 16.2259) (221.616, 16.3058) (221.7492, 16.4656) knots 0 0 0 0 1 1 1 1
  spline S40 degree 3 poles (221.7492, 16.4656) (221.8912, 16.6343) (221.9889, 16.8961) (222.0421, 17.2512) knots 0 0 0 0 1 1 1 1
  line L4 (222.0421, 17.2512) -> (222.1619, 18.0767)
  spline S41 degree 3 poles (222.1619, 18.0767) (221.3276, 17.6062) (220.9104, 17.1491) (220.9104, 16.7053) knots 0 0 0 0 1 1 1 1
  spline S42 degree 3 poles (230.3642, 24.8672) (230.5684, 25.0803) (230.8169, 25.1868) (231.1099, 25.1868) knots 0 0 0 0 1 1 1 1
  spline S43 degree 3 poles (231.1099, 25.1868) (231.4028, 25.1868) (231.6513, 25.0803) (231.8555, 24.8672) knots 0 0 0 0 1 1 1 1
  spline S44 degree 3 poles (231.8555, 24.8672) (232.0685, 24.6631) (232.1751, 24.4145) (232.1751, 24.1216) knots 0 0 0 0 1 1 1 1
  spline S45 degree 3 poles (232.1751, 24.1216) (232.1751, 23.8287) (232.0685, 23.5801) (231.8555, 23.376) knots 0 0 0 0 1 1 1 1
  spline S46 degree 3 poles (231.8555, 23.376) (231.6513, 23.1718) (231.4028, 23.0697) (231.1099, 23.0697) knots 0 0 0 0 1 1 1 1
  spline S47 degree 3 poles (231.1099, 23.0697) (230.8169, 23.0697) (230.5684, 23.1718) (230.3642, 23.376) knots 0 0 0 0 1 1 1 1
  spline S48 degree 3 poles (230.3642, 23.376) (230.1601, 23.5801) (230.058, 23.8287) (230.058, 24.1216) knots 0 0 0 0 1 1 1 1
  spline S49 degree 3 poles (230.058, 24.1216) (230.058, 24.4145) (230.1601, 24.6631) (230.3642, 24.8672) knots 0 0 0 0 1 1 1 1
  spline S50 degree 3 poles (229.8183, 20.966) (229.9071, 21.1258) (230.0758, 21.2456) (230.3243, 21.3255) knots 0 0 0 0 1 1 1 1
  spline S51 degree 3 poles (230.3243, 21.3255) (230.5728, 21.4143) (230.8169, 21.4586) (231.0566, 21.4586) knots 0 0 0 0 1 1 1 1
  spline S52 degree 3 poles (231.0566, 21.4586) (231.3051, 21.4586) (231.5226, 21.4276) (231.709, 21.3654) knots 0 0 0 0 1 1 1 1
  spline S53 degree 3 poles (231.709, 21.3654) (231.3629, 18.6936) (231.1898, 17.3444) (231.1898, 17.3178) knots 0 0 0 0 1 1 1 1
  spline S54 degree 3 poles (231.1898, 17.3178) (231.1454, 17.1402) (231.1232, 16.9893) (231.1232, 16.8651) knots 0 0 0 0 1 1 1 1
  spline S55 degree 3 poles (231.1232, 16.8651) (231.1232, 16.7497) (231.1321, 16.6476) (231.1498, 16.5588) knots 0 0 0 0 1 1 1 1
  spline S56 degree 3 poles (231.1498, 16.5588) (231.1853, 16.328) (231.3451, 16.2126) (231.6291, 16.2126) knots 0 0 0 0 1 1 1 1
  spline S57 degree 3 poles (231.6291, 16.2126) (231.9221, 16.2126) (232.1884, 16.399) (232.428, 16.7719) knots 0 0 0 0 1 1 1 1
  spline S58 degree 3 poles (232.428, 16.7719) (232.6766, 17.1535) (232.863, 17.584) (232.9873, 18.0634) knots 0 0 0 0 1 1 1 1
  spline S59 degree 3 poles (232.9873, 18.0634) (233.0494, 18.0279) (233.147, 17.9214) (233.2802, 17.7438) knots 0 0 0 0 1 1 1 1
  spline S60 degree 3 poles (233.2802, 17.7438) (233.4133, 17.5663) (233.4932, 17.4332) (233.5198, 17.3444) knots 0 0 0 0 1 1 1 1
  spline S61 degree 3 poles (233.5198, 17.3444) (233.3423, 16.6343) (233.0405, 16.0617) (232.6144, 15.6268) knots 0 0 0 0 1 1 1 1
  spline S62 degree 3 poles (232.6144, 15.6268) (232.1884, 15.1918) (231.678, 14.9744) (231.0832, 14.9744) knots 0 0 0 0 1 1 1 1
  spline S63 degree 3 poles (231.0832, 14.9744) (230.4885, 14.9744) (230.0447, 15.1208) (229.7518, 15.4137) knots 0 0 0 0 1 1 1 1
  spline S64 degree 3 poles (229.7518, 15.4137) (229.4677, 15.7067) (229.3257, 16.0839) (229.3257, 16.5455) knots 0 0 0 0 1 1 1 1
  spline S65 degree 3 poles (229.3257, 16.5455) (229.3257, 16.6431) (229.3301, 16.7452) (229.339, 16.8517) knots 0 0 0 0 1 1 1 1
  line L5 (229.339, 16.8517) -> (229.8183, 20.966)
  spline S66 degree 3 poles (235.4431, 24.3346) (235.4431, 24.2814) (235.3232, 23.3272) (235.0836, 21.472) knots 0 0 0 0 1 1 1 1
  line L6 (235.0836, 21.472) -> (237.0408, 21.472)
  line L7 (237.0408, 21.472) -> (237.0408, 20.4467)
  line L8 (237.0408, 20.4467) -> (234.9504, 20.4467)
  line L9 (234.9504, 20.4467) -> (234.9105, 20.1139)
  spline S67 degree 3 poles (234.9105, 20.1139) (235.949, 19.244) (236.4683, 18.2942) (236.4683, 17.2645) knots 0 0 0 0 1 1 1 1
  spline S68 degree 3 poles (236.4683, 17.2645) (236.4683, 16.4567) (236.2597, 15.8753) (235.8425, 15.5203) knots 0 0 0 0 1 1 1 1
  spline S69 degree 3 poles (235.8425, 15.5203) (235.4342, 15.1652) (234.9416, 14.9877) (234.3646, 14.9877) knots 0 0 0 0 1 1 1 1
  spline S70 degree 3 poles (234.3646, 14.9877) (233.7876, 14.9877) (233.366, 15.1386) (233.0997, 15.4404) knots 0 0 0 0 1 1 1 1
  spline S71 degree 3 poles (233.0997, 15.4404) (232.8334, 15.7511) (232.7002, 16.1239) (232.7002, 16.5588) knots 0 0 0 0 1 1 1 1
  spline S72 degree 3 poles (232.7002, 16.5588) (232.7002, 16.6564) (232.7091, 16.763) (232.7269, 16.8784) knots 0 0 0 0 1 1 1 1
  line L10 (232.7269, 16.8784) -> (233.1396, 20.4201)
  line L11 (233.1396, 20.4201) -> (233.0864, 20.4467)
  line L12 (233.0864, 20.4467) -> (232.0079, 20.4467)
  spline S73 degree 3 poles (232.0079, 20.4467) (231.999, 20.5355) (231.9946, 20.6775) (231.9946, 20.8728) knots 0 0 0 0 1 1 1 1
  spline S74 degree 3 poles (231.9946, 20.8728) (231.9946, 21.077) (232.0345, 21.2767) (232.1144, 21.472) knots 0 0 0 0 1 1 1 1
  line L13 (232.1144, 21.472) -> (233.2595, 21.472)
  line L14 (233.2595, 21.472) -> (233.6855, 25.0936)
  spline S75 degree 3 poles (233.6855, 25.0936) (233.8719, 25.1646) (234.1205, 25.2001) (234.4312, 25.2001) knots 0 0 0 0 1 1 1 1
  spline S76 degree 3 poles (234.4312, 25.2001) (235.1058, 25.2001) (235.4431, 24.9116) (235.4431, 24.3346) knots 0 0 0 0 1 1 1 1
  spline S77 degree 3 poles (235.5762, 17.2778) (235.5762, 17.8903) (235.3099, 18.4939) (234.7773, 19.0886) knots 0 0 0 0 1 1 1 1
  spline S78 degree 3 poles (234.7773, 19.0886) (234.6176, 17.766) (234.5377, 17.0027) (234.5377, 16.7985) knots 0 0 0 0 1 1 1 1
  spline S79 degree 3 poles (234.5377, 16.7985) (234.5377, 16.399) (234.6664, 16.1993) (234.9238, 16.1993) knots 0 0 0 0 1 1 1 1
  spline S80 degree 3 poles (234.9238, 16.1993) (235.1102, 16.1993) (235.2656, 16.2837) (235.3898, 16.4523) knots 0 0 0 0 1 1 1 1
  spline S81 degree 3 poles (235.3898, 16.4523) (235.5141, 16.6298) (235.5762, 16.905) (235.5762, 17.2778) knots 0 0 0 0 1 1 1 1
  spline S82 degree 3 poles (240.0201, 24.3346) (240.0201, 24.2814) (239.9002, 23.3272) (239.6606, 21.472) knots 0 0 0 0 1 1 1 1
  line L15 (239.6606, 21.472) -> (241.6178, 21.472)
  line L16 (241.6178, 21.472) -> (241.6178, 20.4467)
  line L17 (241.6178, 20.4467) -> (239.5274, 20.4467)
  line L18 (239.5274, 20.4467) -> (239.4875, 20.1139)
  spline S83 degree 3 poles (239.4875, 20.1139) (240.526, 19.244) (241.0453, 18.2942) (241.0453, 17.2645) knots 0 0 0 0 1 1 1 1
  spline S84 degree 3 poles (241.0453, 17.2645) (241.0453, 16.4567) (240.8366, 15.8753) (240.4195, 15.5203) knots 0 0 0 0 1 1 1 1
  spline S85 degree 3 poles (240.4195, 15.5203) (240.0111, 15.1652) (239.5185, 14.9877) (238.9416, 14.9877) knots 0 0 0 0 1 1 1 1
  spline S86 degree 3 poles (238.9416, 14.9877) (238.3646, 14.9877) (237.9429, 15.1386) (237.6766, 15.4404) knots 0 0 0 0 1 1 1 1
  spline S87 degree 3 poles (237.6766, 15.4404) (237.4103, 15.7511) (237.2772, 16.1239) (237.2772, 16.5588) knots 0 0 0 0 1 1 1 1
  spline S88 degree 3 poles (237.2772, 16.5588) (237.2772, 16.6564) (237.2861, 16.763) (237.3038, 16.8784) knots 0 0 0 0 1 1 1 1
  line L19 (237.3038, 16.8784) -> (237.7166, 20.4201)
  line L20 (237.7166, 20.4201) -> (237.6633, 20.4467)
  line L21 (237.6633, 20.4467) -> (236.5848, 20.4467)
  spline S89 degree 3 poles (236.5848, 20.4467) (236.576, 20.5355) (236.5715, 20.6775) (236.5715, 20.8728) knots 0 0 0 0 1 1 1 1
  spline S90 degree 3 poles (236.5715, 20.8728) (236.5715, 21.077) (236.6114, 21.2767) (236.6913, 21.472) knots 0 0 0 0 1 1 1 1
  line L22 (236.6913, 21.472) -> (237.8364, 21.472)
  line L23 (237.8364, 21.472) -> (238.2625, 25.0936)
  spline S91 degree 3 poles (238.2625, 25.0936) (238.4489, 25.1646) (238.6974, 25.2001) (239.0081, 25.2001) knots 0 0 0 0 1 1 1 1
  spline S92 degree 3 poles (239.0081, 25.2001) (239.6826, 25.2001) (240.0201, 24.9116) (240.0201, 24.3346) knots 0 0 0 0 1 1 1 1
  spline S93 degree 3 poles (240.1532, 17.2778) (240.1532, 17.8903) (239.8869, 18.4939) (239.3543, 19.0886) knots 0 0 0 0 1 1 1 1
  spline S94 degree 3 poles (239.3543, 19.0886) (239.1945, 17.766) (239.1147, 17.0027) (239.1147, 16.7985) knots 0 0 0 0 1 1 1 1
  spline S95 degree 3 poles (239.1147, 16.7985) (239.1147, 16.399) (239.2432, 16.1993) (239.5008, 16.1993) knots 0 0 0 0 1 1 1 1
  spline S96 degree 3 poles (239.5008, 16.1993) (239.6872, 16.1993) (239.8424, 16.2837) (239.9668, 16.4523) knots 0 0 0 0 1 1 1 1
  spline S97 degree 3 poles (239.9668, 16.4523) (240.091, 16.6298) (240.1532, 16.905) (240.1532, 17.2778) knots 0 0 0 0 1 1 1 1
  spline S98 degree 3 poles (244.0643, 18.0501) (244.6148, 18.1655) (245.023, 18.3874) (245.2893, 18.7158) knots 0 0 0 0 1 1 1 1
  spline S99 degree 3 poles (245.2893, 18.7158) (245.5645, 19.0442) (245.702, 19.3594) (245.702, 19.6611) knots 0 0 0 0 1 1 1 1
  spline S100 degree 3 poles (245.702, 19.6611) (245.702, 19.9718) (245.6178, 20.1804) (245.449, 20.2869) knots 0 0 0 0 1 1 1 1
  spline S101 degree 3 poles (245.449, 20.2869) (245.2893, 20.4023) (245.1118, 20.46) (244.9165, 20.46) knots 0 0 0 0 1 1 1 1
  spline S102 degree 3 poles (244.9165, 20.46) (244.4993, 20.46) (244.1309, 20.2248) (243.8113, 19.7544) knots 0 0 0 0 1 1 1 1
  spline S103 degree 3 poles (243.8113, 19.7544) (243.5007, 19.2928) (243.3453, 18.738) (243.3453, 18.09) knots 0 0 0 0 1 1 1 1
  spline S104 degree 3 poles (243.3453, 18.09) (243.3453, 17.4509) (243.4963, 16.9716) (243.798, 16.652) knots 0 0 0 0 1 1 1 1
  spline S105 degree 3 poles (243.798, 16.652) (244.1088, 16.3413) (244.4904, 16.186) (244.9431, 16.186) knots 0 0 0 0 1 1 1 1
  spline S106 degree 3 poles (244.9431, 16.186) (245.6088, 16.186) (246.2479, 16.4168) (246.8604, 16.8784) knots 0 0 0 0 1 1 1 1
  spline S107 degree 3 poles (246.8604, 16.8784) (247.4729, 17.34) (247.9701, 17.9435) (248.3517, 18.6892) knots 0 0 0 0 1 1 1 1
  spline S108 degree 3 poles (248.3517, 18.6892) (248.547, 18.5028) (248.7245, 18.272) (248.8842, 17.9968) knots 0 0 0 0 1 1 1 1
  spline S109 degree 3 poles (248.8842, 17.9968) (248.5913, 17.3311) (248.072, 16.6786) (247.3264, 16.0395) knots 0 0 0 0 1 1 1 1
  spline S110 degree 3 poles (247.3264, 16.0395) (246.9536, 15.7289) (246.5098, 15.4759) (245.9949, 15.2806) knots 0 0 0 0 1 1 1 1
  spline S111 degree 3 poles (245.9949, 15.2806) (245.489, 15.0853) (244.9653, 14.9877) (244.4238, 14.9877) knots 0 0 0 0 1 1 1 1
  spline S112 degree 3 poles (244.4238, 14.9877) (243.5363, 14.9877) (242.835, 15.2584) (242.3201, 15.7999) knots 0 0 0 0 1 1 1 1
  spline S113 degree 3 poles (242.3201, 15.7999) (241.7698, 16.3857) (241.4946, 17.1358) (241.4946, 18.0501) knots 0 0 0 0 1 1 1 1
  spline S114 degree 3 poles (241.4946, 18.0501) (241.4946, 18.9644) (241.8364, 19.7632) (242.5198, 20.4467) knots 0 0 0 0 1 1 1 1
  spline S115 degree 3 poles (242.5198, 20.4467) (243.2122, 21.1302) (244.0377, 21.472) (244.9963, 21.472) knots 0 0 0 0 1 1 1 1
  spline S116 degree 3 poles (244.9963, 21.472) (245.68, 21.472) (246.2346, 21.3211) (246.6607, 21.0193) knots 0 0 0 0 1 1 1 1
  spline S117 degree 3 poles (246.6607, 21.0193) (247.0868, 20.7263) (247.3044, 20.3269) (247.3131, 19.8209) knots 0 0 0 0 1 1 1 1
  spline S118 degree 3 poles (247.3131, 19.8209) (247.3131, 19.1374) (247.0381, 18.5827) (246.4876, 18.1566) knots 0 0 0 0 1 1 1 1
  spline S119 degree 3 poles (246.4876, 18.1566) (245.9463, 17.7305) (245.2006, 17.4332) (244.2507, 17.2645) knots 0 0 0 0 1 1 1 1
  line L24 (244.2507, 17.2645) -> (244.0643, 18.0501)
  spline S120 degree 3 poles (256.7474, 19.8609) (256.7474, 18.9377) (256.1969, 18.232) (255.0963, 17.7438) knots 0 0 0 0 1 1 1 1
  spline S121 degree 3 poles (255.0963, 17.7438) (255.123, 17.584) (255.1629, 17.3932) (255.2162, 17.1713) knots 0 0 0 0 1 1 1 1
  spline S122 degree 3 poles (255.2162, 17.1713) (255.3759, 16.5144) (255.6422, 16.1771) (256.0151, 16.1594) knots 0 0 0 0 1 1 1 1
  spline S123 degree 3 poles (256.0151, 16.1594) (256.0417, 16.1594) (256.0683, 16.1594) (256.0949, 16.1594) knots 0 0 0 0 1 1 1 1
  spline S124 degree 3 poles (256.0949, 16.1594) (256.805, 16.1594) (257.3332, 16.7852) (257.6794, 18.0368) knots 0 0 0 0 1 1 1 1
  spline S125 degree 3 poles (257.6794, 18.0368) (257.8658, 17.8681) (258.0433, 17.6151) (258.212, 17.2778) knots 0 0 0 0 1 1 1 1
  spline S126 degree 3 poles (258.212, 17.2778) (258.0876, 16.7985) (257.9101, 16.3946) (257.6794, 16.0662) knots 0 0 0 0 1 1 1 1
  spline S127 degree 3 poles (257.6794, 16.0662) (257.4574, 15.7377) (257.2134, 15.5025) (256.9471, 15.3605) knots 0 0 0 0 1 1 1 1
  spline S128 degree 3 poles (256.9471, 15.3605) (256.4765, 15.1119) (256.0327, 14.9877) (255.6156, 14.9877) knots 0 0 0 0 1 1 1 1
  spline S129 degree 3 poles (255.6156, 14.9877) (254.6391, 14.9877) (253.9556, 15.5336) (253.5651, 16.6254) knots 0 0 0 0 1 1 1 1
  spline S130 degree 3 poles (253.5651, 16.6254) (253.4141, 17.0603) (253.3122, 17.5042) (253.2589, 17.9569) knots 0 0 0 0 1 1 1 1
  spline S131 degree 3 poles (253.2589, 17.9569) (253.7649, 18.0811) (254.1643, 18.2853) (254.4572, 18.5693) knots 0 0 0 0 1 1 1 1
  spline S132 degree 3 poles (254.4572, 18.5693) (254.7502, 18.8623) (254.8966, 19.1729) (254.8966, 19.5014) knots 0 0 0 0 1 1 1 1
  spline S133 degree 3 poles (254.8966, 19.5014) (254.8966, 20.0695) (254.6124, 20.3535) (254.0445, 20.3535) knots 0 0 0 0 1 1 1 1
  spline S134 degree 3 poles (254.0445, 20.3535) (253.7337, 20.3535) (253.4674, 20.2337) (253.2456, 19.994) knots 0 0 0 0 1 1 1 1
  spline S135 degree 3 poles (253.2456, 19.994) (253.0236, 19.7632) (252.8771, 19.4836) (252.8062, 19.1552) knots 0 0 0 0 1 1 1 1
  spline S136 degree 3 poles (252.8062, 19.1552) (252.7529, 18.7025) (252.6641, 17.9879) (252.5399, 17.0115) knots 0 0 0 0 1 1 1 1
  spline S137 degree 3 poles (252.5399, 17.0115) (252.4244, 16.044) (252.3489, 15.396) (252.3136, 15.0676) knots 0 0 0 0 1 1 1 1
  line L25 (252.3136, 15.0676) -> (250.5427, 15.0676)
  spline S138 degree 3 poles (250.5427, 15.0676) (251.1818, 20.5089) (251.5679, 23.8509) (251.7011, 25.0936) knots 0 0 0 0 1 1 1 1
  spline S139 degree 3 poles (251.7011, 25.0936) (251.8875, 25.1646) (252.1405, 25.2001) (252.46, 25.2001) knots 0 0 0 0 1 1 1 1
  spline S140 degree 3 poles (252.46, 25.2001) (253.1524, 25.2001) (253.4986, 24.9959) (253.4986, 24.5876) knots 0 0 0 0 1 1 1 1
  line L26 (253.4986, 24.5876) -> (253.4986, 24.5077)
  spline S141 degree 3 poles (253.4986, 24.5077) (253.3209, 22.9011) (253.1568, 21.6717) (253.0059, 20.8195) knots 0 0 0 0 1 1 1 1
  spline S142 degree 3 poles (253.0059, 20.8195) (253.494, 21.2722) (254.1065, 21.4986) (254.8434, 21.4986) knots 0 0 0 0 1 1 1 1
  spline S143 degree 3 poles (254.8434, 21.4986) (255.3936, 21.4986) (255.8463, 21.3566) (256.2015, 21.0725) knots 0 0 0 0 1 1 1 1
  spline S144 degree 3 poles (256.2015, 21.0725) (256.5653, 20.7885) (256.7474, 20.3846) (256.7474, 19.8609) knots 0 0 0 0 1 1 1 1
  spline S145 degree 3 poles (259.7976, 18.0501) (260.3479, 18.1655) (260.7562, 18.3874) (261.0225, 18.7158) knots 0 0 0 0 1 1 1 1
  spline S146 degree 3 poles (261.0225, 18.7158) (261.2978, 19.0442) (261.4353, 19.3594) (261.4353, 19.6611) knots 0 0 0 0 1 1 1 1
  spline S147 degree 3 poles (261.4353, 19.6611) (261.4353, 19.9718) (261.351, 20.1804) (261.1823, 20.2869) knots 0 0 0 0 1 1 1 1
  spline S148 degree 3 poles (261.1823, 20.2869) (261.0225, 20.4023) (260.8451, 20.46) (260.6497, 20.46) knots 0 0 0 0 1 1 1 1
  spline S149 degree 3 poles (260.6497, 20.46) (260.2326, 20.46) (259.8642, 20.2248) (259.5446, 19.7544) knots 0 0 0 0 1 1 1 1